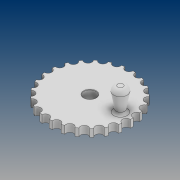
# Autodesk Inventor part: 10_Banh_lai
Saved by Autodesk Inventor 2021 (Build 250183000, 183)
## iProperties
Created: 2024-04-09
Part Number: 10_Banh_lai
Material: Generic
Document SubType Name: Modeling
Designer: Admin
Density: 1 g/cm^3
Appearance: Default
Author: Admin
Autodesk Inventor part; units mm, degrees
ref_plane "YZ Plane" through (0, 0, 0) normal (1, 0, 0) x (0, 1, 0)
ref_plane "XZ Plane" through (0, 0, 0) normal (0, 1, 0) x (-1, 0, 0)
ref_plane "XY Plane" through (0, 0, 0) normal (0, 0, 1) x (1, 0, 0)
sketch "Sketch1" plane through (0, 0, 0) normal (0, 1, 0) x (-1, 0, 0)
  circle A0 centre (0, 0) radius 3.9
  circle A1 centre (0, 0) radius 35.5
  circle A2 centre (0, 0) radius 27.5
  circle A3 centre (0, 0) radius 8.9
  circle A4 centre (27.5, 0) radius 2.5
  line L0 (27.5, 0) -> (0, 0)
  circle A5 centre (26.636, 6.839) radius 2.5
  circle A6 centre (24.0984, 13.2482) radius 2.5
  circle A7 centre (20.0466, 18.825) radius 2.5
  circle A8 centre (14.7352, 23.219) radius 2.5
  circle A9 centre (8.498, 26.1541) radius 2.5
  circle A10 centre (1.7267, 27.4457) radius 2.5
  circle A11 centre (-5.153, 27.0129) radius 2.5
  circle A12 centre (-11.7089, 24.8827) radius 2.5
  circle A13 centre (-17.5292, 21.1891) radius 2.5
  circle A14 centre (-22.248, 16.1641) radius 2.5
  circle A15 centre (-25.5689, 10.1234) radius 2.5
  circle A16 centre (-27.2832, 3.4467) radius 2.5
  circle A17 centre (-27.2832, -3.4467) radius 2.5
  circle A18 centre (-25.5689, -10.1234) radius 2.5
  circle A19 centre (-22.248, -16.1641) radius 2.5
  circle A20 centre (-17.5292, -21.1891) radius 2.5
  circle A21 centre (-11.7089, -24.8827) radius 2.5
  circle A22 centre (-5.153, -27.0129) radius 2.5
  circle A23 centre (1.7267, -27.4457) radius 2.5
  circle A24 centre (8.498, -26.1541) radius 2.5
  circle A25 centre (14.7352, -23.219) radius 2.5
  circle A26 centre (20.0466, -18.825) radius 2.5
  circle A27 centre (24.0984, -13.2482) radius 2.5
  circle A28 centre (26.636, -6.839) radius 2.5
  point P0 (27.3864, 2.4974)
  point P1 (27.1471, 4.3918)
  point P2 (25.9049, 9.2297)
  point P3 (25.202, 11.005)
  point P4 (22.7957, 15.382)
  point P5 (21.6734, 16.9267)
  point P6 (18.2542, 20.5678)
  point P7 (16.783, 21.7849)
  point P8 (12.5657, 24.4613)
  point P9 (10.838, 25.2742)
  point P10 (6.0877, 26.8177)
  point P11 (4.2121, 27.1755)
  point P12 (-0.7729, 27.4891)
  point P13 (-2.6785, 27.3692)
  point P14 (-7.5849, 26.4333)
  point P15 (-9.4008, 25.8433)
  point P16 (-13.9203, 23.7166)
  point P17 (-15.5324, 22.6935)
  point P18 (-19.381, 19.5096)
  point P19 (-20.6881, 18.1178)
  point P20 (-23.624, 14.0768)
  point P21 (-24.5438, 12.4036)
  point P22 (-26.3826, 7.7596)
  point P23 (-26.8574, 5.9101)
  point P24 (-27.4834, 0.9547)
  point P25 (-27.4834, -0.9547)
  point P26 (-26.8574, -5.9101)
  point P27 (-26.3826, -7.7596)
  point P28 (-24.5438, -12.4036)
  point P29 (-23.624, -14.0768)
  point P30 (-20.6881, -18.1178)
  point P31 (-19.381, -19.5096)
  point P32 (-15.5324, -22.6935)
  point P33 (-13.9203, -23.7166)
  point P34 (-9.4008, -25.8433)
  point P35 (-7.5849, -26.4333)
  point P36 (-2.6785, -27.3692)
  point P37 (-0.7729, -27.4891)
  point P38 (4.2121, -27.1755)
  point P39 (6.0877, -26.8177)
  point P40 (10.838, -25.2742)
  point P41 (12.5657, -24.4613)
  point P42 (16.783, -21.7849)
  point P43 (18.2542, -20.5678)
  point P44 (21.6734, -16.9267)
  point P45 (22.7957, -15.382)
  point P46 (25.202, -11.005)
  point P47 (25.9049, -9.2297)
  point P48 (27.1471, -4.3918)
  point P49 (27.3864, -2.4974)
  dimension "d3" = 55
  dimension "d0" = 7.8
  dimension "d1" = 5
  dimension "d4" = 5
  dimension "d7" = 360
  dimension "d13" = 8
  constraints: 28 centre point, 3 coincident, 2 end point, 1 horizontal, 54 other
  measures "d0" diameter of A0
  measures "d1" radial gap between concentric circles of A0 A3
  measures "d4" diameter of A4
extrude "Extrusion1" add sketch "Sketch1" along normal blind 5 contours A4 A2 A28 A27 A26 A25 A24 A23 A22 A21 A20 A19 A18 A17 A16 A15 A14 A13 A12 A11 A10 A9 A8 A7 A6 A5 | A3
extrude "Extrusion2" add sketch "Sketch1" against normal blind 5 contours A3
sketch "Sketch2" plane through (0, 0, 0) normal (1, 0, 0) x (0, 1, 0)
  line L0 (-5, 8.9) -> (-5, -8.9) projected
  line L1 (0, -8.9) -> (0, 8.9) projected
  circle A0 centre (-2.5, 0) radius 1.4
  point P0 (0, 0)
  dimension "d14" = 2.5
  dimension "d17" = 2.8
  constraints: 1 centre point
  measures "d14" distance from line of L0 A0.centre
  measures "d17" diameter of A0
extrude "Extrusion3" cut sketch "Sketch2" along normal blind 10.5
pattern_circular "Circular Pattern1" count 2 over 90 about axis through (0, 0, 0) along (0, -1, 0) of "Extrusion3"
fillet "Fillet1" radius 0.25 3 edges at (8.9, -5, 0) (3.9, -5, 0) (3.9, 5, 0)
sketch "Sketch3" plane through (0, 5, 0) normal (0, 1, 0) x (1, 0, 0)
  circle A0 centre (20, 0) radius 2.5
  point P0 (0, 0)
  dimension "d22" = 20
  dimension "d23" = 5
  constraints: 1 centre point
  measures "d22" distance of point (0, 0) A0.centre
  measures "d23" diameter of A0
ref_plane "Work Plane1" through (0, 20, 0) normal (0, 1, 0) x (1, 0, 0)
sketch "Sketch4" plane through (0, 20, 0) normal (0, 1, 0) x (1, 0, 0)
  circle A0 centre (20, 0) radius 2.5 construction
  circle A1 centre (20, 0) radius 5
  point P0 (0, 0)
  dimension "d25" = 10
  constraints: 1 centre point, 1 coincident
  measures "d25" diameter of A1
loft "Loft1" add profiles "Sketch4", "Sketch3"
fillet "Fillet2" radius 1.5 1 edges at (17.5, 5, 0)
fillet "Fillet3" radius 2.75 1 edges at (15, 20, 0)
body "Solid1"
